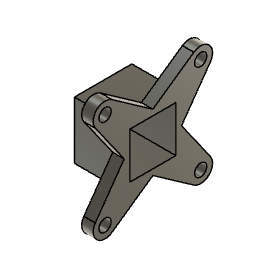
Motor-mainrod fitting v1.2 (Autodesk Fusion 360 design; units mm, degrees)
Autodesk Fusion 360 part; units mm, degrees
sketch "Sketch1" plane through (0, 0, 0) normal (1, 0, 0) x (0, 1, 0)
  line L0 (9.5131, 10.735) -> (-5.4869, 10.735)
  line L1 (-5.4869, 10.735) -> (-5.4869, -4.265)
  line L2 (-5.4869, -4.265) -> (9.5131, -4.265)
  line L3 (9.5131, -4.265) -> (9.5131, 10.735)
  line L4 (9.5131, 10.735) -> (-5.4869, -4.265) construction
  line L5 (-5.4869, 10.735) -> (9.5131, -4.265) construction
  line L6 (8.0131, -2.765) -> (-3.9869, -2.765)
  line L7 (-3.9869, -2.765) -> (-3.9869, 9.235)
  line L8 (-3.9869, 9.235) -> (8.0131, 9.235)
  line L9 (8.0131, 9.235) -> (8.0131, -2.765)
  line L10 (8.0131, -2.765) -> (-3.9869, 9.235) construction
  line L11 (-3.9869, -2.765) -> (8.0131, 9.235) construction
  point P0 (2.0131, 3.235)
  point P1 (2.0131, 3.235)
  dimension "d3" = 15
  dimension "d4" = 15
  dimension "d5" = 12
  dimension "d6" = 12
  constraint horizontal L0
  constraint perpendicular L0 L1
  constraint parallel L0 L2
  constraint parallel L1 L3
  constraint coincident L4 P1
  constraint coincident L5 P1
  constraint horizontal L6
  constraint perpendicular L6 L7
  constraint parallel L6 L8
  constraint parallel L7 L9
  constraint coincident L10 P1
  constraint coincident L11 P1
  constraint coincident P1 P0
  measures "d3" distance of L1.end L2.end
  measures "d4" distance of L0.end L1.end
  measures "d5" distance of L7.end L8.end
  measures "d6" distance of L6.end L7.end
extrude "Extrude1" add sketch "Sketch1" along normal blind 5
sketch "Sketch2" plane through (5, 0, 0) normal (1, 0, 0) x (0, 1, 0)
  line L0 (-3.9869, 9.235) -> (8.0131, 9.235)
  line L1 (8.0131, 9.235) -> (8.0131, -2.765)
  line L2 (8.0131, -2.765) -> (-3.9869, -2.765)
  line L3 (-3.9869, -2.765) -> (-3.9869, 9.235)
  line L4 (9.5131, -4.265) -> (9.5131, 10.735)
  line L5 (9.5131, 10.735) -> (-5.4869, 10.735)
  line L6 (-5.4869, 10.735) -> (-5.4869, -4.265)
  line L7 (-5.4869, -4.265) -> (9.5131, -4.265)
  line L8 (17.0131, 18.235) -> (-12.9869, -11.765) construction
  line L9 (-12.9869, 18.235) -> (17.0131, -11.765) construction
  circle A0 centre (14.5131, 15.735) radius 1.6
  circle A1 centre (-10.4869, 15.735) radius 1.6
  circle A2 centre (-10.4869, -9.265) radius 1.6
  circle A3 centre (14.5131, -9.265) radius 1.6
  circle A4 centre (-10.4869, 15.735) radius 3.1
  circle A5 centre (14.5131, 15.735) radius 3.1
  circle A6 centre (-10.4869, -9.265) radius 3.1
  line L10 (9.5131, 10.735) -> (-5.4869, 10.735)
  line L11 (-5.4869, 10.735) -> (-5.4869, -4.265)
  line L12 (-5.4869, -4.265) -> (9.5131, -4.265)
  line L13 (9.5131, -4.265) -> (9.5131, 10.735)
  line L14 (9.5131, 10.735) -> (-5.4869, -4.265) construction
  line L15 (-5.4869, 10.735) -> (9.5131, -4.265) construction
  line L16 (-8.7038, 18.2708) -> (2.0131, 10.735)
  line L17 (2.0131, 10.735) -> (12.73, 18.2708)
  line L18 (-13.0227, 13.9519) -> (-5.4869, 3.235)
  line L19 (-5.4869, 3.235) -> (-13.0227, -7.4819)
  line L20 (-8.7038, -11.8008) -> (2.0131, -4.265)
  line L21 (9.5131, 3.235) -> (17.0489, 13.9519)
  circle A7 centre (14.5131, -9.265) radius 3.1
  line L22 (9.5131, 3.235) -> (17.0489, -7.4819)
  line L23 (2.0131, -4.265) -> (12.73, -11.8008)
  point P0 (2.0131, 3.235)
  point P1 (2.0131, 3.235)
  point P2 (2.0131, 3.235)
  dimension "d11" = 3.2
  dimension "d12" = 12.5
  dimension "d13" = 3.2
  dimension "d14" = 3.2
  dimension "d15" = 3.2
  dimension "d17" = 25
  dimension "d18" = 12.5
  dimension "d19" = 25
  dimension "d20" = 6.2
  dimension "d21" = 6.2
  dimension "d22" = 6.2
  dimension "d23" = 6.2
  constraint coincident L8 P2
  constraint coincident L9 P2
  constraint coincident P2 P1
  constraint horizontal A0.centre A1.centre
  constraint vertical A1.centre A2.centre
  constraint horizontal A2.centre A3.centre
  constraint vertical A0.centre A3.centre
  constraint concentric A1 A4
  constraint concentric A0 A5
  constraint concentric A2 A6
  constraint horizontal L10
  constraint perpendicular L10 L11
  constraint parallel L10 L12
  constraint parallel L11 L13
  constraint coincident L14 P2
  constraint coincident L15 P2
  constraint coincident L4.end L5.start
  constraint coincident A4 L16.start
  constraint midpoint L10 L16.end
  constraint tangent A4 L16
  constraint coincident A5 L17.end
  constraint tangent A5 L17
  constraint coincident A4 L18.start
  constraint midpoint L11 L18.end
  constraint coincident A6 L19.end
  constraint tangent A6 L19
  constraint tangent A4 L18
  constraint coincident A6 L20.start
  constraint midpoint L12 L20.end
  constraint tangent A6 L20
  constraint midpoint L13 L21.start
  constraint coincident A5 L21.end
  constraint tangent A5 L21
  constraint concentric A3 A7
  constraint coincident A7 L22.end
  constraint tangent A7 L22
  constraint coincident A7 L23.end
  constraint tangent A7 L23
  measures "d11" diameter of A0
  measures "d12" horizontal distance of P2 A0.centre
  measures "d13" diameter of A1
  measures "d14" diameter of A2
  measures "d15" diameter of A3
  measures "d17" horizontal distance of A0.centre A1.centre
  measures "d18" vertical distance of P2 A0.centre
  measures "d19" vertical distance of A0.centre A3.centre
  measures "d20" diameter of A4
  measures "d21" diameter of A5
  measures "d22" diameter of A6
  measures "d23" diameter of A7
extrude "Extrude2" add sketch "Sketch2" along normal blind 3
extrude "Extrude4" add sketch "Sketch1" against normal blind 5
extrude "Extrude3" [suppressed]
equation "d11 = motorScrewHole"
equation "d13 = motorScrewHole"
equation "d14 = motorScrewHole"
equation "d15 = motorScrewHole"
equation "motorScrewHole = 3.2 mm" comment "poo"
equation "d20 = motorScrewHole + 3 mm"
equation "d21 = motorScrewHole + 3 mm"
equation "d22 = motorScrewHole + 3 mm"
equation "d23 = motorScrewHole + 3 mm"
